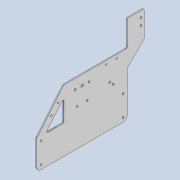
# Autodesk Inventor part: X Axis V Wheel RIGHT Outside Frame Machined
Saved by Autodesk Inventor 2022 (Build 260153000, 153)
## iProperties
Created: 2021-10-10
Part Number: X Axis V Wheel RIGHT Outside Frame Machined
Material: Generic
Document SubType Name: Modeling
Designer: Coy
Density: 1 g/cm^3
Appearance: Machined - Aluminum
Author: Coy
Autodesk Inventor part; units mm, degrees
ref_plane "YZ Plane" through (0, 0, 0) normal (1, 0, 0) x (0, 1, 0)
ref_plane "XZ Plane" through (0, 0, 0) normal (0, 1, 0) x (-1, 0, 0)
ref_plane "XY Plane" through (0, 0, 0) normal (0, 0, 1) x (1, 0, 0)
sketch "Sketch1" plane through (0, 0, 0) normal (1, 0, 0) x (0, 1, 0)
  line L0 (-120.8333, -99.25) -> (-47.8333, -99.25)
  line L1 (-120.2, -86.75) -> (-120.2, -99.25) construction
  line L2 (0, -198.5) -> (40, -198.5) construction
  line L3 (40, -198.5) -> (40, -265) construction
  line L4 (40, -265) -> (0, -265) construction
  line L5 (0, -265) -> (0, -198.5) construction
  line L6 (0, -265) -> (40, -265) construction
  line L7 (40, -265) -> (40, -285) construction
  line L8 (40, -285) -> (0, -285)
  line L9 (0, -285) -> (0, -265) construction
  line L10 (0, -198.5) -> (40, -198.5) construction
  line L11 (40, -198.5) -> (40, -178.5) construction
  line L12 (40, -178.5) -> (0, -178.5) construction
  line L13 (0, -178.5) -> (0, -198.5) construction
  line L14 (48.2, -259.95) -> (-8.2, -259.95) construction
  line L15 (-8.2, -259.95) -> (-8.2, -203.55) construction
  line L16 (-8.2, -203.55) -> (48.2, -203.55) construction
  line L17 (48.2, -203.55) -> (48.2, -259.95) construction
  line L18 (48.2, -231.75) -> (-8.2, -231.75) construction
  line L19 (40, -231.75) -> (0, -231.75) construction
  line L20 (43.57, -255.32) -> (-3.57, -255.32) construction
  line L21 (-3.57, -255.32) -> (-3.57, -208.18) construction
  line L22 (-3.57, -208.18) -> (43.57, -208.18) construction
  line L23 (43.57, -208.18) -> (43.57, -255.32) construction
  line L24 (43.57, -255.32) -> (48.2, -255.32) construction
  line L25 (43.57, -255.32) -> (43.57, -259.95) construction
  line L26 (-3.57, -208.18) -> (-8.2, -208.18) construction
  line L27 (-3.57, -208.18) -> (-3.57, -203.55) construction
  line L28 (40, -188.5) -> (0, -188.5) construction
  line L29 (40, -275) -> (0, -275) construction
  circle A0 centre (30, -275) radius 2.1
  circle A1 centre (10, -275) radius 2.1
  circle A2 centre (30, -188.5) radius 2.1
  circle A3 centre (10, -188.5) radius 2.1
  circle A4 centre (43.57, -255.32) radius 2.6
  circle A5 centre (43.57, -208.18) radius 2.6
  circle A6 centre (-3.57, -208.18) radius 2.6
  circle A7 centre (-3.57, -255.32) radius 2.6
  circle A8 centre (20, -231.75) radius 19.15
  circle A9 centre (-25, -216.75) radius 11.08 construction
  circle A10 centre (-25, -216.75) radius 13 construction
  circle A11 centre (-25, -216.75) radius 2.5
  line L30 (-60, -351.75) -> (-60, -111.75) construction
  circle A12 centre (-60, -111.75) radius 2.6
  circle A13 centre (-60, -351.75) radius 2.6
  line L31 (-120.2, -351.75) -> (-120.2, -111.75) construction
  circle A14 centre (-120.2, -111.75) radius 2.6
  circle A15 centre (-120.2, -351.75) radius 2.6
  circle A16 centre (-60, -111.75) radius 12 construction
  circle A17 centre (-120.2, -111.75) radius 12 construction
  circle A18 centre (-120.2, -351.75) radius 12 construction
  circle A19 centre (-60, -351.75) radius 12 construction
  circle A20 centre (-25, -246.75) radius 2.5
  circle A21 centre (-25, -246.75) radius 11.08 construction
  circle A22 centre (-25, -246.75) radius 13 construction
  circle A23 centre (20, -231.75) radius 11.08 construction
  circle A24 centre (20, -231.75) radius 13 construction
  line L32 (-23.1873, -227.6807) -> (18.1873, -220.8193) construction
  line L33 (18.1873, -242.6807) -> (-23.1873, -235.8193) construction
  line L34 (-47.8333, -364.25) -> (-120.8333, -364.25)
  line L35 (-132.8333, -352.25) -> (-132.8333, -111.25)
  line L36 (-60, -351.75) -> (-120.2, -351.75) construction
  line L37 (-120.2, -111.75) -> (-60, -111.75) construction
  line L38 (-60, -351.75) -> (-60, -364.25) construction
  line L39 (-120.2, -111.75) -> (-120.2, -99.25) construction
  line L40 (48.3276, -178.5) -> (48.3276, -285)
  line L41 (17.6122, -285) -> (40, -285) construction
  arc A25 (-132.8333, -352.25) -> (-120.8333, -364.25) centre (-120.8333, -352.25) ccw
  arc A26 (-120.8333, -99.25) -> (-132.8333, -111.25) centre (-120.8333, -111.25) ccw
  line L42 (48.3276, -178.5) -> (-47.8333, -99.25)
  line L43 (-47.8333, -364.25) -> (-47.8333, -99.25) construction
  line L44 (-120.2, -111.75) -> (-132.8333, -111.75) construction
  line L45 (-60, -351.75) -> (-47.8333, -351.75) construction
  line L46 (-36.08, -246.75) -> (-36.08, -485.113) construction
  line L47 (-47.8333, -344.25) -> (-47.8333, -285)
  line L48 (-47.8333, -285) -> (16.8804, -285)
  line L49 (-47.8333, -125.1668) -> (16.8804, -178.5)
  line L50 (-47.8333, -178.5) -> (16.8804, -178.5)
  line L51 (-47.8333, -125.1668) -> (-47.8333, -178.5)
  line L52 (48.3276, -285) -> (48.3276, -364.25)
  line L53 (48.3276, -364.25) -> (-47.8333, -364.25)
  line L54 (-47.8333, -344.25) -> (28.3276, -344.25)
  line L55 (28.3276, -344.25) -> (28.3276, -285)
  line L56 (-47.8333, -344.25) -> (28.3276, -285) construction
  line L57 (-39.6904, -344.25) -> (28.3276, -291.3349)
  line L58 (-47.8333, -337.9151) -> (20.1847, -285)
  line L59 (48.3276, -414.25) -> (124.3276, -414.25)
  line L60 (124.3276, -414.25) -> (124.3276, -364.25)
  line L61 (124.3276, -364.25) -> (48.3276, -364.25)
  line L62 (48.3276, -364.25) -> (48.3276, -414.25)
  line L63 (48.3276, -414.25) -> (-1.6724, -364.25)
  line L64 (98.3276, -364.25) -> (48.3276, -314.25)
  point P0 (-132.8333, -99.25)
  point P1 (28.3276, 86.5)
  point P2 (0, 86.5)
  point P3 (20.1847, 86.5)
  point P4 (20.1847, 86.5)
  point P5 (0, 86.5)
  point P6 (-132.8333, -364.25)
  point P7 (-47.8333, -338.3332)
  point P8 (0, -285)
  point P9 (48.3276, -364.25)
  dimension "d222" = 85
  dimension "d242" = 76
  dimension "d243" = 50
  dimension "d244" = 45
  dimension "d245" = 50
  dimension "d246" = 45
  constraints: 130 end point, 29 point on line, 26 centre point, 18 coincident, 8 point on circle, 2 horizontal, 2 parallel, 2 perpendicular, 1 collinear, 1 symmetric about line, 3 other
  measures "d222" distance of L0.end point (-132.833, -99.25)
  measures "d242" distance of L61.end L60.end
  measures "d243" distance of L60.end L59.end
  measures "d244" angle of L62 L63
  measures "d245" distance from line of L62 L64.start
  measures "d246" angle of L61 L64
extrude "Extrusion1" add sketch "Sketch1" along normal blind 3.175 contours L0 L42 L40 L52 L53 L34 A25 L35 A26 | L62 L63 L53 | L61 L60 L59 L62 | L55 L57 L54 L47 L58 L8 | L58 L47 L48 L8 | L55 L54 L57 | A0 | A1 | A2 | A3 | A4 | A5 | A6 | A7 | A8
sketch "Sketch6" plane through (3.175, 0, 0) normal (1, 0, 0) x (0, 0, -1)
  line L0 (125.1668, -47.8333) -> (178.5, 16.8804) projected
  line L1 (291.3349, 28.3276) -> (344.25, 28.3276) projected
  line L2 (159.4204, -6.2705) -> (143.9864, 6.4492) construction
  line L3 (178.5, 48.3276) -> (99.25, -47.8333) construction
  line L4 (291.3349, 28.3276) -> (344.25, 28.3276) construction
  line L5 (317.7924, 28.3276) -> (317.7924, 48.3276) construction
  line L6 (364.25, 48.3276) -> (178.5, 48.3276) construction
  line L7 (151.7034, 0.0893) -> (161.2432, 11.6648) construction
  line L8 (151.7034, 0.0893) -> (142.1636, -11.4861) construction
  line L9 (317.7924, 38.3276) -> (302.7924, 38.3276) construction
  line L10 (317.7924, 38.3276) -> (332.7924, 38.3276) construction
  circle A0 centre (332.7924, 38.3276) radius 2.6
  circle A1 centre (302.7924, 38.3276) radius 2.6
  circle A2 centre (161.2432, 11.6648) radius 2.6
  circle A3 centre (142.1636, -11.4861) radius 2.6
  point P0 (414.25, 48.3276)
  point P1 (314.25, 48.3276)
  dimension "d233" = 15
  dimension "d234" = 15
  dimension "d235" = 15
  dimension "d236" = 15
  dimension "d237" = 5.2
  dimension "d238" = 5.2
  dimension "d239" = 5.2
  dimension "d240" = 5.2
  dimension "d241" = 30
  constraints: 12 end point, 5 perpendicular, 4 centre point, 4 coincident, 3 midpoint, 3 point on line, 1 vertical
  measures "d233" distance of L7.start L7.end
  measures "d234" distance of L7.start L8.end
  measures "d235" distance of L9.start L9.end
  measures "d236" distance of L9.start L10.end
  measures "d237" diameter of A0
  measures "d238" diameter of A1
  measures "d239" diameter of A2
  measures "d240" diameter of A3
  measures "d241" distance from line of L0.end L2
extrude "Extrusion6" cut sketch "Sketch6" against normal through all
fillet "Fillet2" radius 3.175 5 edges at (1.5875, -47.8333, -125.1668) (1.5875, -47.8333, -178.5) (1.5875, 16.8804, -178.5) (1.5875, -47.8333, -99.25) (1.5875, 48.3276, -178.5)
fillet "Fillet3" radius 3.175 5 edges at (1.5875, 48.3276, -364.25) (1.5875, -1.6724, -364.25) (1.5875, 48.3276, -414.25) (1.5875, 124.3276, -414.25) (1.5875, 124.3276, -364.25)
sketch "Sketch7" plane through (3.175, 0, 0) normal (1, 0, 0) x (0, 0, -1)
  line L0 (414.25, 49.6427) -> (414.25, 121.1526) construction
  line L1 (414.25, 121.5776) -> (394.25, 121.5776) construction
  line L2 (394.25, 121.5776) -> (394.25, 71.5776) construction
  line L3 (394.25, 71.5776) -> (414.25, 71.5776) construction
  line L4 (414.25, 71.5776) -> (414.25, 121.5776) construction
  line L5 (404.25, 121.5776) -> (404.25, 71.5776) construction
  circle A0 centre (404.25, 106.5776) radius 2.6
  circle A1 centre (404.25, 86.5776) radius 2.6
  line L6 (411.075, 124.3276) -> (367.425, 124.3276) projected
  point P0 (0, 0)
  dimension "d248" = 20
  dimension "d249" = 50
  dimension "d250" = 5.2
  dimension "d251" = 5.2
  dimension "d252" = 15
  dimension "d253" = 15
  dimension "d256" = 2.75
  constraints: 10 end point, 3 point on line, 2 centre point, 2 midpoint, 2 parallel, 1 horizontal, 1 perpendicular
  measures "d248" distance of L3.end L2.end
  measures "d249" distance of L2.end L1.end
  measures "d250" diameter of A0
  measures "d251" diameter of A1
  measures "d252" distance from line of L1 A0.centre
  measures "d253" distance from line of L3 A1.centre
  measures "d256" distance between parallel lines of L6 L1
extrude "Extrusion7" cut sketch "Sketch7" against normal up to next
sketch "Sketch8" plane through (3.175, 0, 0) normal (1, 0, 0) x (0, 0, -1)
  line L0 (302.7924, 28.3276) -> (332.7924, 28.3276) construction
  line L1 (332.7924, 28.3276) -> (332.7924, -26.6724) construction
  line L2 (332.7924, -26.6724) -> (302.7924, -26.6724) construction
  line L3 (302.7924, -26.6724) -> (302.7924, 28.3276) construction
  circle A0 centre (332.7924, 38.3276) radius 2.6 projected
  circle A1 centre (302.7924, 38.3276) radius 2.6 projected
  line L4 (332.7924, 38.3276) -> (302.7924, 38.3276) construction
  line L5 (317.7924, 38.3276) -> (317.7924, 28.3276) construction
  line L6 (328.7924, -26.6724) -> (306.7924, -26.6724) construction
  line L7 (306.7924, -26.6724) -> (306.7924, -6.6724) construction
  line L8 (306.7924, -6.6724) -> (328.7924, -6.6724) construction
  line L9 (328.7924, -6.6724) -> (328.7924, -26.6724) construction
  line L10 (312.7924, -11.6724) -> (322.7924, -11.6724) construction
  line L11 (322.7924, -11.6724) -> (322.7924, -21.6724) construction
  line L12 (322.7924, -21.6724) -> (312.7924, -21.6724) construction
  line L13 (312.7924, -21.6724) -> (312.7924, -11.6724) construction
  circle A2 centre (312.7924, -11.6724) radius 2.6
  circle A3 centre (322.7924, -21.6724) radius 2.6
  point P0 (0, 0)
  dimension "d257" = 30
  dimension "d258" = 55
  dimension "d259" = 10
  dimension "d260" = 22
  dimension "d261" = 20
  dimension "d262" = 4
  dimension "d263" = 10
  dimension "d264" = 10
  dimension "d265" = 5
  dimension "d266" = 6
  dimension "d267" = 5.2
  dimension "d268" = 5.2
  constraints: 28 end point, 6 parallel, 4 horizontal, 4 perpendicular, 2 centre point, 2 coincident, 2 midpoint, 1 point on line
  measures "d257" distance of L1.end L2.end
  measures "d258" distance of L0.end L1.end
  measures "d259" distance of L5.start L5.end
  measures "d260" distance of L7.end L8.end
  measures "d261" distance of L6.end L7.end
  measures "d262" distance between parallel lines of L3 L7
  measures "d263" distance of L11.end L12.end
  measures "d264" distance of L10.end L11.end
  measures "d265" distance between parallel lines of L8 L10
  measures "d266" distance between parallel lines of L7 L13
  measures "d267" diameter of A2
  measures "d268" diameter of A3
extrude "Extrusion8" cut sketch "Sketch8" against normal up to next contours A2 | A3
sketch "Sketch9" plane through (3.175, 0, 0) normal (1, 0, 0) x (0, 0, -1)
  line L0 (45.8374, 19.9996) -> (577.1226, 19.9996) construction
  line L1 (361.075, 48.3276) -> (179.9977, 48.3276) construction
  line L2 (231.7502, 111.484) -> (231.7502, -169.9488) construction
  circle A0 centre (161.2432, 11.6648) radius 2.6 projected
  circle A1 centre (231.7502, 19.9996) radius 3.5
  circle A2 centre (251.7502, 19.9996) radius 2.6
  circle A3 centre (211.7502, 19.9996) radius 2.6
  point P0 (0, 0)
  dimension "d271" = 28.328
  dimension "d272" = 70.507
  dimension "d273" = 7
  dimension "d274" = 5.2
  dimension "d275" = 20
  dimension "d276" = 5.2
  dimension "d277" = 20
  constraints: 4 end point, 4 point on line, 3 centre point, 1 horizontal, 1 vertical
  measures "d271" distance between parallel lines of L1 L0
  measures "d272" distance from line of A0.centre L2
  measures "d273" diameter of A1
  measures "d274" diameter of A2
  measures "d275" distance of A1.centre A2.centre
  measures "d276" diameter of A3
  measures "d277" distance of A1.centre A3.centre
extrude "Extrusion9" cut sketch "Sketch9" against normal up to next contours A1 | A2 | A3
body "Solid1"
